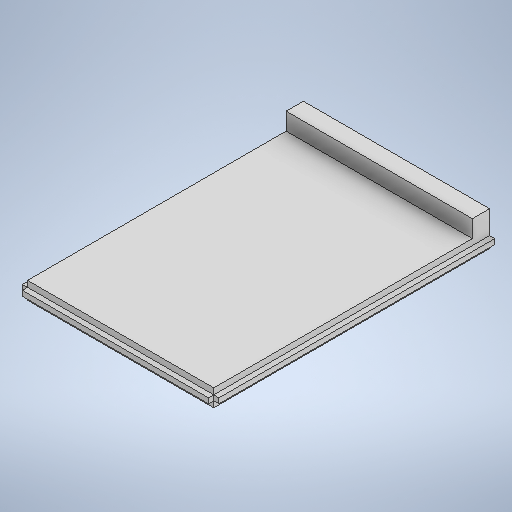
# Autodesk Inventor part: couvercle pilier
Saved by Autodesk Inventor 2025.2 (Build 292293000, 293)
## iProperties
Created: 2026-03-19
Part Number: couvercle pilier
Material: Générique
Document SubType Name: Modeling
Designer: rphilipped
Density: 1 g/cm^3
Appearance: Par défaut
Author: rphilipped
Autodesk Inventor part; units mm, degrees
ref_plane "YZ Plane" through (0, 0, 0) normal (1, 0, 0) x (0, 1, 0)
ref_plane "XZ Plane" through (0, 0, 0) normal (0, 1, 0) x (-1, 0, 0)
ref_plane "XY Plane" through (0, 0, 0) normal (0, 0, 1) x (1, 0, 0)
sketch "Esquisse1" plane through (0, 0, 0) normal (0, 1, 0) x (-1, 0, 0)
  line L0 (0, 0) -> (108, 0)
  line L1 (108, 0) -> (108, -160)
  line L2 (108, -160) -> (0, -160)
  line L3 (0, -160) -> (0, 0)
  dimension "d0" = 108
  dimension "d1" = 160
  constraints: 8 end point, 2 parallel, 1 horizontal, 1 perpendicular
  measures "d0" distance of L1.end L2.end
  measures "d1" distance of L0.end L1.end
extrude "Extrusion1" add sketch "Esquisse1" along normal blind 10
sketch "Esquisse2" plane through (0, 10, 0) normal (0, 1, 0) x (1, 0, 0)
  line L0 (0, 160) -> (-108, 160) projected
  line L1 (-108, 160) -> (-108, 0) projected
  line L2 (0, 160) -> (-108, 160)
  line L3 (-108, 160) -> (-108, 150)
  line L4 (-108, 150) -> (0, 150)
  line L5 (0, 150) -> (0, 160)
  point P0 (0, 0)
  dimension "d4" = 10
  constraints: 8 end point, 2 parallel, 1 horizontal, 1 perpendicular, 1 point on line
  measures "d4" distance of L4.end L0.start
extrude "Extrusion2" add sketch "Esquisse2" along normal blind 10
sketch "Esquisse3" plane through (0, 0, 0) normal (0, -1, 0) x (1, 0, 0)
  line L0 (-44, -142.4556) -> (-64, -142.4556)
  line L1 (0, 0) -> (0, -160) projected
  line L2 (-108, -160) -> (-108, 0) projected
  line L3 (-54, -122.4556) -> (-64, -142.4556)
  line L4 (-54, -122.4556) -> (-44, -142.4556)
  dimension "d7" = 20
  dimension "d8" = 44
  dimension "d9" = 44
  constraints: 6 end point, 1 horizontal
  measures "d7" distance of L0.start L0.end
  measures "d8" distance from line of L1 L0.start
  measures "d9" distance from line of L2 L0.end
extrude "Extrusion3" cut sketch "Esquisse3" against normal blind 5
sketch "Esquisse4" plane through (-108, 0, -160) normal (-1, 0, 0) x (0, 0, 1)
  line L0 (0, 0) -> (0, 20) projected
  line L1 (0, 6.5) -> (160, 6.5)
  line L2 (160, 0) -> (0, 0) projected
  line L3 (160, 6.5) -> (160, 3.5)
  line L4 (160, 3.5) -> (0, 3.5)
  line L5 (17.5444, 5) -> (37.5444, 5) projected
  line L6 (0, 3.5) -> (0, 6.5)
  point P0 (0, 3.5)
  dimension "d13" = 3
  dimension "d14" = 3.5
  constraints: 8 end point, 2 parallel, 2 perpendicular, 1 point on line
  measures "d13" distance of L1.end L3.end
  measures "d14" distance between parallel lines of L4 L2
extrude "Extrusion4" add sketch "Esquisse4" along normal blind 3
sketch "Esquisse5" plane through (0, 0, 0) normal (1, 0, 0) x (0, 0, -1)
  line L0 (0, 3.5) -> (160, 3.5) projected
  line L1 (0, 3.5) -> (160, 3.5)
  line L2 (160, 6.5) -> (0, 6.5) projected
  line L3 (160, 3.5) -> (160, 6.5)
  line L4 (160, 6.5) -> (160, 3.5)
  line L5 (0, 6.5) -> (160, 6.5)
  line L6 (0, 6.5) -> (0, 3.5)
  line L7 (0, 0) -> (0, 10) projected
  constraints: 10 end point, 2 collinear, 2 perpendicular, 1 parallel
extrude "Extrusion5" add sketch "Esquisse5" along normal blind 3
sketch "Esquisse6" plane through (-108, 0, 0) normal (0, 0, 1) x (1, 0, 0)
  line L0 (0, 6.5) -> (-3, 6.5) projected
  line L1 (108, 6.5) -> (108, 10) projected
  line L2 (0, 6.5) -> (108, 6.5)
  line L3 (0, 3.5) -> (-3, 3.5) projected
  line L4 (108, 3.5) -> (0, 3.5)
  line L5 (0, 6.5) -> (0, 10) projected
  line L6 (0, 6.5) -> (0, 3.5)
  line L7 (108, 6.5) -> (108, 3.5)
  point P0 (108, 0)
  constraints: 8 end point, 1 horizontal, 1 perpendicular, 1 vertical
extrude "Extrusion6" add sketch "Esquisse6" along normal blind 3
